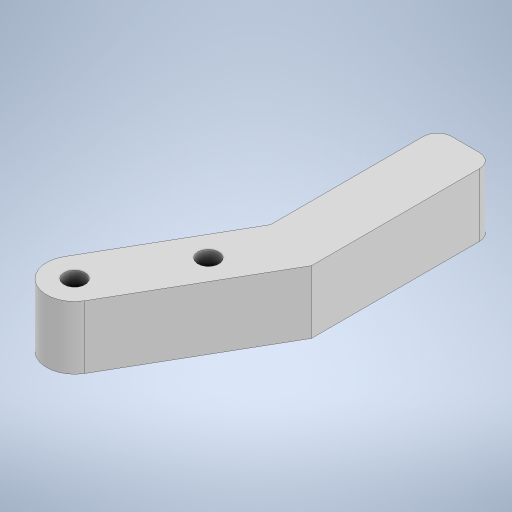
# Autodesk Inventor part: Pinza_pieza3
Saved by Autodesk Inventor 2023 (Build 270158000, 158)
## iProperties
Created: 2024-09-28
Part Number: Pinza_pieza3
Material: Genérico
Document SubType Name: Sheet Metal
Designer: sebas
Density: 1 g/cm^3
Sheet Metal Rule: Por defecto_mm
Appearance: Valor por defecto
Author: sebas
Autodesk Inventor part; units mm, degrees
ref_plane "YZ Plane" through (0, 0, 0) normal (1, 0, 0) x (0, 1, 0)
ref_plane "XZ Plane" through (0, 0, 0) normal (0, 1, 0) x (-1, 0, 0)
ref_plane "XY Plane" through (0, 0, 0) normal (0, 0, 1) x (1, 0, 0)
sketch "Boceto1" plane through (0, 0, 0) normal (0, 1, 0) x (-1, 0, 0)
  line L0 (0, 2) -> (0, 26)
  line L1 (0, 26) -> (11.8564, 46.5359)
  line L2 (17.3205, 48) -> (17.3205, 48)
  line L3 (18.7846, 42.5359) -> (8, 23.8564)
  line L4 (8, 23.8564) -> (8, 2)
  line L5 (6, 0) -> (2, 0)
  arc A0 (81.7987, 0) -> (84.2987, 9.3301) centre (81.7987, 5) ccw
  arc A1 (18.7846, 42.5359) -> (17.3205, 48) centre (15.3205, 44.5359) ccw
  arc A2 (17.3205, 48) -> (11.8564, 46.5359) centre (15.3205, 44.5359) ccw
  arc A3 (6, 0) -> (8, 2) centre (6, 2) ccw
  arc A4 (0, 2) -> (2, 0) centre (2, 2) ccw
  circle A5 centre (15.3205, 44.5359) radius 1.5
  line L6 (15.3205, 44.5359) -> (4.5694, 25.9145) construction
  circle A6 centre (8.3205, 32.4115) radius 1.5
  point P0 (0, 0)
  point P1 (13.8564, 50)
  point P2 (8, 0)
  point P3 (20.7846, 46)
  point P4 (4, 0)
  dimension "d0" = 90
  dimension "d2" = 26
  dimension "d7" = 8
  dimension "d10" = 150
  dimension "d11" = 8
  dimension "d12" = 5
  dimension "d13" = 4
  dimension "d14" = 4
  dimension "d15" = 2
  dimension "d16" = 3
  dimension "d17" = 3
  dimension "d18" = 14
  dimension "d19" = 48
  constraints: 14 end point, 10 point on circle, 10 point on line, 10 tangent, 7 centre point, 2 parallel, 2 perpendicular, 1 coincident, 1 equal radius, 1 midpoint, 1 vertical
  measures "d0" angle of L1 L2
  measures "d2" distance of point (0, 0) L0.end
  measures "d7" distance of point (20.785, 46) point (13.856, 50)
  measures "d10" angle of L1 L0
  measures "d11" distance of point (8, 0) point (0, 0)
  measures "d12" radius of A0
  measures "d13" radius of A1
  measures "d14" radius of A2
  measures "d15" radius of A3
  measures "d16" diameter of A5
  measures "d17" diameter of A6
  measures "d18" distance of A6.centre A2.centre
  measures "d19" vertical distance of point (4, 0) L2.end
extrude "Extrusión1" add sketch "Boceto1" along normal mid plane 9
equation "\"Radio_pliegue\" = Grosor"
equation "\"Anchura_desahogo_plegado\" = Grosor"
equation "\"Profundidad_desahogo_plegado\" = 0.5 * Grosor"
equation "\"Tamaño_destalonado\" = 4 * Grosor"
equation "\"Remanente_mínimo\" = 2 * Grosor"
equation "\"Radiodetransición\" = Radio_pliegue"
equation "\"Tamaño_de_radio_de_Jacobi\" = Radio_pliegue"
equation "\"TamañoSeparación\" = Grosor"
equation "\"Grosor\" = 0.5"
